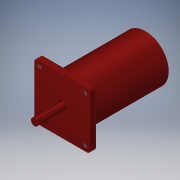
# Autodesk Inventor part: 12V DC Motor
Saved by Autodesk Inventor 2019 (Build 230136000, 136)
## iProperties
Created: 2020-01-10
Part Number: 12V DC Motor
Material: Stainless Steel, Polished
Document SubType Name: Modeling
Designer: 18186
Density: 8 g/cm^3
Appearance: Anodized - Red
Author: 18186
Autodesk Inventor part; units mm, degrees
ref_plane "YZ Plane" through (0, 0, 0) normal (1, 0, 0) x (0, 1, 0)
ref_plane "XZ Plane" through (0, 0, 0) normal (0, 1, 0) x (-1, 0, 0)
ref_plane "XY Plane" through (0, 0, 0) normal (0, 0, 1) x (1, 0, 0)
sketch "Sketch1" plane through (0, 0, 0) normal (0, 0, 1) x (1, 0, 0)
  line L0 (-27.305, -30.48) -> (27.305, -30.48)
  line L1 (30.48, -27.305) -> (30.48, 27.305)
  line L2 (27.305, 30.48) -> (-27.305, 30.48)
  line L3 (-30.48, 27.305) -> (-30.48, -27.305)
  line L4 (-30.48, -30.48) -> (30.48, 30.48) construction
  line L5 (30.48, -30.48) -> (-30.48, 30.48) construction
  arc A0 (-27.305, 30.48) -> (-30.48, 27.305) centre (-27.305, 27.305) ccw
  arc A1 (-30.48, -27.305) -> (-27.305, -30.48) centre (-27.305, -27.305) ccw
  arc A2 (30.48, 27.305) -> (27.305, 30.48) centre (27.305, 27.305) ccw
  arc A3 (27.305, -30.48) -> (30.48, -27.305) centre (27.305, -27.305) ccw
  point P0 (0, 0)
  dimension "d0" = 60.96
  dimension "d1" = 60.96
  dimension "d2" = 3.175
  constraints: 12 end point, 8 point on circle, 8 point on line, 8 tangent, 4 centre point, 3 equal radius, 2 midpoint, 2 parallel, 1 horizontal, 1 perpendicular
  measures "d0" distance of L5.end L4.end
  measures "d1" distance of L4.end L5.start
  measures "d2" radius of A0
extrude "Extrusion1" add sketch "Sketch1" along normal blind 6.35
sketch "Sketch2" plane through (0, 0, 6.35) normal (0, 0, 1) x (1, 0, 0)
  arc A0 (-27.305, 30.48) -> (-30.48, 27.305) centre (-27.305, 27.305) ccw projected
  arc A1 (30.48, 27.305) -> (27.305, 30.48) centre (27.305, 27.305) ccw projected
  arc A2 (27.305, -30.48) -> (30.48, -27.305) centre (27.305, -27.305) ccw projected
  arc A3 (-30.48, -27.305) -> (-27.305, -30.48) centre (-27.305, -27.305) ccw projected
  line L0 (-27.305, 27.305) -> (27.305, -27.305) construction
  line L1 (-27.305, -27.305) -> (27.305, 27.305) construction
  point P0 (0, 0)
  point P1 (-25.0599, 25.0599)
  point P2 (25.0599, 25.0599)
  point P3 (25.0599, -25.0599)
  point P4 (-25.0599, -25.0599)
  constraints: 4 end point, 4 point on line
hole "Hole1" at (-25.0599, 25.0599, 6.35) at (25.0599, 25.0599, 6.35) at (25.0599, -25.0599, 6.35) at (-25.0599, -25.0599, 6.35) direction (0, 0, -1) diameter 4.9784 end through all thread size "1/4-20 UNC" class "2B" standard "ANSI Unified Screw Threads"
sketch "Sketch3" plane through (0, 0, 0) normal (0, 0, -1) x (-1, 0, 0)
  circle A0 centre (0, 0) radius 25.4
  dimension "d12" = 50.8
  constraints: 1 centre point, 1 coincident
  measures "d12" diameter of A0
extrude "Extrusion2" add sketch "Sketch3" along normal blind 85.09
sketch "Sketch4" plane through (0, 0, 6.35) normal (0, 0, 1) x (1, 0, 0)
  circle A0 centre (0, 0) radius 5.08
  dimension "d15" = 10.16
  constraints: 1 centre point, 1 coincident
  measures "d15" diameter of A0
extrude "Extrusion3" cut sketch "Sketch4" against normal blind 50.8
sketch "Sketch5" plane through (0, 0, -44.45) normal (0, 0, 1) x (1, 0, 0)
  circle A0 centre (0, 0) radius 3.81
  dimension "d18" = 7.62
  constraints: 1 centre point, 1 coincident
  measures "d18" diameter of A0
extrude "Extrusion4" add sketch "Sketch5" along normal blind 81.28
body "Solid1"
